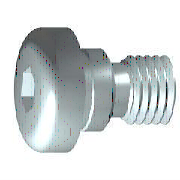
# Autodesk Inventor part: 100005
Saved by Autodesk Inventor 2020.1 (Build 241239000, 239)
## iProperties
Created: 2006-01-26
Part Number: 100005
Material: Steel, Mild
Description: Hexagon socket head shoulder screws
Document SubType Name: Modeling
Standard: ISO  7379
Designer: Kevin
Standard Revision: First edition 1983-10-01
Standards Organization: ISO
Language: en-US
Size Designation: 8  x 30
Categories: <MemberInstance><Categories><Category DisplayName="Fasteners" InternalName="e4da775c-781d-43d5-af7c-5136215cf5a6" Mnemonic="FSTN"><Category DisplayName="Bolts" InternalName="536e6df0-f778-49ac-b2f2-25c71d2aa0b2" Mnemonic="SCRW"><CategoryParameter DisplayName="Nominal Diameter" InternalName="8bbe3f8e-44cf-40a9-a251-3a6edc8168d6" Mnemonic="nomdia"/><CategoryParameter DisplayName="Nominal Length" InternalName="238ecbaf-3e6c-45dd-aa95-4068c8e0fd02" Mnemonic="nomlen"/><CategoryParameter DisplayName="Thread Series Designation" InternalName="87c5849c-b3a5-4c3e-9c9b-2feecef9be86" Mnemonic="thrserdsgn"/><CategoryParameter DisplayName="Thread Class" InternalName="ebc0d23b-2cc6-4d2a-b376-d52aae53bab6" Mnemonic="thrclss"/><CategoryParameter DisplayName="Thread Designation" InternalName="586d5e89-370a-4089-914f-0110033585c7" Mnemonic="thrdesign"/><CategoryParameter DisplayName="Thread Type" InternalName="b4bbb7bc-d6aa-4c9f-a9a9-4152b9f6fe49" Mnemonic="thrtype"/><CategoryParameter DisplayName="Threads per Unit" InternalName="bdc6e7d2-ffd0-4d9c-a173-16b95ebb912d" Mnemonic="thrperunit1"/><CategoryParameter DisplayName="Thread Pitch" InternalName="bb82302e-82d8-4176-8fc1-c5d7bb17d5ad" Mnemonic="pitch1"/><CategoryParameter DisplayName="Nominal Diameter Designation" InternalName="03caf894-eafd-4c09-a035-916ac084b87b" Mnemonic="nomdiadesig"/><Category DisplayName="Socket Head" InternalName="55e06bf3-7e58-486c-bbdc-745fcc60664d" Mnemonic="CLSCRW"><CategoryParameter DisplayName="Shank Diameter" InternalName="179dbae3-102f-48bb-85fe-1e3ecd34f7cc" Mnemonic="grpdia"/><CategoryParameter DisplayName="Grip Length" InternalName="52eab69f-422f-4795-9995-175a1b827e67" Mnemonic="grplen"/><CategoryParameter DisplayName="Thread Length" InternalName="3268731d-5f9a-4750-8b01-4a959c46fbf2" Mnemonic="thrlen"/><CategoryParameter DisplayName="Head Diameter" InternalName="46177176-dbdd-4a1b-aefd-4c60c45016af" Mnemonic="headdia"/><CategoryParameter DisplayName="Head Height" InternalName="99c92c4c-4a02-4ebe-9e64-948fb169e19e" Mnemonic="headh"/><CategoryParameter DisplayName="Type" InternalName="59a7e495-7a0c-4a5c-bdfd-c090c5f6e2db" Mnemonic="type"/><Category DisplayName="Shoulder" InternalName="90bdf7a4-4d26-46b5-8948-baa3e50baddb" Mnemonic="FTCLSCREW"><CategoryParameter DisplayName="Shank Length" InternalName="fd35b191-8e29-43b8-8902-775fde943ca0" Mnemonic="shnklen"/><CategoryParameter DisplayName="Shank Diameter" InternalName="3f11206c-57b2-4a53-88eb-c02e573d836e" Mnemonic="grpdia"/></Category></Category></Category></Category></Categories><FamilyTemplate Id="nf0093"><FamilyTemplateParameters><FamilyTemplateParameter ObjectType="kUserParameterObject" ValueType="xs:double" Id="1" ObjectReferenceKey="KOD"/><FamilyTemplateParameter ObjectType="kUserParameterObject" ValueType="xs:double" Id="2" ObjectReferenceKey="BDMM"/><FamilyTemplateParameter ObjectType="kUserParameterObject" ValueType="xs:double" Id="3" ObjectReferenceKey="FAWI3"/><FamilyTemplateParameter ObjectType="kUserParameterObject" ValueType="xs:double" Id="4" ObjectReferenceKey="FAWI2"/><FamilyTemplateParameter ObjectType="kUserParameterObject" ValueType="xs:double" Id="5" ObjectReferenceKey="BDM"/><FamilyTemplateParameter ObjectType="kUserParameterObject" ValueType="xs:double" Id="6" ObjectReferenceKey="SW"/><FamilyTemplateParameter ObjectType="kUserParameterObject" ValueType="xs:double" Id="7" ObjectReferenceKey="FAWI4"/><FamilyTemplateParameter ObjectType="kUserParameterObject" ValueType="xs:double" Id="8" ObjectReferenceKey="PTC"/><FamilyTemplateParameter ObjectType="kUserParameterObject" ValueType="xs:double" Id="9" ObjectReferenceKey="NLG"/><FamilyTemplateParameter ObjectType="kUserParameterObject" ValueType="xs:double" Id="10" ObjectReferenceKey="LOTI"/><FamilyTemplateParameter ObjectType="kUserParameterObject" ValueType="xs:double" Id="11" ObjectReferenceKey="BOR"/><FamilyTemplateParameter ObjectType="kUserParameterObject" ValueType="xs:double" Id="12" ObjectReferenceKey="GUL"/><FamilyTemplateParameter ObjectType="kUserParameterObject" ValueType="xs:double" Id="13" ObjectReferenceKey="SLG"/><FamilyTemplateParameter ObjectType="kUserParameterObject" ValueType="xs:double" Id="14" ObjectReferenceKey="THREADDIA"/><FamilyTemplateParameter ObjectType="kUserParameterObject" ValueType="xs:double" Id="15" ObjectReferenceKey="E0"/><FamilyTemplateParameter ObjectType="kUserParameterObject" ValueType="xs:double" Id="16" ObjectReferenceKey="TPU"/><FamilyTemplateParameter ObjectType="kUserParameterObject" ValueType="xs:double" Id="17" ObjectReferenceKey="TOA"/><FamilyTemplateParameter ObjectType="kUserParameterObject" ValueType="xs:double" Id="18" ObjectReferenceKey="SPD"/><FamilyTemplateParameter ObjectType="kUserParameterObject" ValueType="xs:double" Id="19" ObjectReferenceKey="PHH"/><FamilyTemplateParameter ObjectType="kUserParameterObject" ValueType="xs:double" Id="20" ObjectReferenceKey="ANG"/><FamilyTemplateParameter ObjectType="kUserParameterObject" ValueType="xs:double" Id="21" ObjectReferenceKey="NND"/><FamilyTemplateParameter ObjectType="kUserParameterObject" ValueType="xs:double" Id="22" ObjectReferenceKey="GD1"/><FamilyTemplateParameter ObjectType="kUserParameterObject" ValueType="xs:double" Id="23" ObjectReferenceKey="GEL"/><FamilyTemplateParameter ObjectType="kUserParameterObject" ValueType="xs:double" Id="24" ObjectReferenceKey="INTI"/><FamilyTemplateParameter ObjectType="kUserParameterObject" ValueType="xs:double" Id="25" ObjectReferenceKey="GAL2"/><FamilyTemplateParameter ObjectType="kUserParameterObject" ValueType="xs:double" Id="26" ObjectReferenceKey="GAL"/><FamilyTemplateParameter ObjectType="kUserParameterObject" ValueType="xs:double" Id="27" ObjectReferenceKey="KOH"/><FamilyTemplateParameter ObjectType="kPropertyObject" ValueType="xs:string" Id="100" ObjectReferenceKey="{32853F0F-3444-11D1-9E93-0060B03C1CA6}" SubObjectId="52"/><FamilyTemplateParameter ObjectType="kPropertyObject" ValueType="xs:string" Id="101" ObjectReferenceKey="{32853F0F-3444-11D1-9E93-0060B03C1CA6}" SubObjectId="49"/><FamilyTemplateParameter ObjectType="kPropertyObject" ValueType="xs:string" Id="102" ObjectReferenceKey="{32853F0F-3444-11D1-9E93-0060B03C1CA6}" SubObjectId="37"/><FamilyTemplateParameter ObjectType="kPropertyObject" ValueType="xs:string" Id="103" ObjectReferenceKey="{32853F0F-3444-11D1-9E93-0060B03C1CA6}" SubObjectId="47"/><FamilyTemplateParameter ObjectType="kPropertyObject" ValueType="xs:string" Id="104" ObjectReferenceKey="{32853F0F-3444-11D1-9E93-0060B03C1CA6}" SubObjectId="48"/><FamilyTemplateParameter ObjectType="kPropertyObject" ValueType="xs:string" Id="105" ObjectReferenceKey="{32853F0F-3444-11D1-9E93-0060B03C1CA6}" SubObjectId="5"/><FamilyTemplateParameter ObjectType="kPropertyObject" ValueType="xs:string" Id="106" ObjectReferenceKey="{32853F0F-3444-11D1-9E93-0060B03C1CA6}" SubObjectId="29"/><FamilyTemplateParameter ObjectType="kPropertyObject" ValueType="xs:string" Id="107" ObjectReferenceKey="{32853F0F-3444-11D1-9E93-0060B03C1CA6}" SubObjectId="20"/><FamilyTemplateParameter ObjectType="kPropertyObject" ValueType="xs:string" Id="108" ObjectReferenceKey="{B9600981-DEE8-4547-8D7C-E525B3A1727A}" SubObjectId="17"/><FamilyTemplateParameter ObjectType="kPropertyObject" ValueType="xs:string" Id="109" ObjectReferenceKey="{B9600981-DEE8-4547-8D7C-E525B3A1727A}" SubObjectId="19"/><FamilyTemplateParameter ObjectType="kPropertyObject" ValueType="xs:string" Id="110" ObjectReferenceKey="{B9600981-DEE8-4547-8D7C-E525B3A1727A}" SubObjectId="21"/><FamilyTemplateParameter ObjectType="kPropertyObject" ValueType="xs:string" Id="111" ObjectReferenceKey="{B9600981-DEE8-4547-8D7C-E525B3A1727A}" SubObjectId="9"/><FamilyTemplateParameter ObjectType="kPartDocumentObject" ValueType="xs:string" Id="112" ObjectReferenceKey="" SubObjectId="DisplayName"/><FamilyTemplateParameter ObjectType="kThreadFeatureObject" ValueType="xs:structure" Id="300" ObjectReferenceKey="1002000010000000e30a0000000000008000000000000000" SubObjectId="ThreadInfo"><FamilyTemplateParameter ValueType="xs:string" Id="301" SubObjectId="ThreadClass"/><FamilyTemplateParameter ValueType="xs:string" Id="302" SubObjectId="ThreadDesignation"/><FamilyTemplateParameter ValueType="xs:string" Id="303" SubObjectId="ThreadType"/></FamilyTemplateParameter><FamilyTemplateParameter ObjectType="kPartFeatureObject" ValueType="xs:string" Id="400" ObjectReferenceKey="10020000100000009f070000000000008000000000000000" SubObjectId="Name"/><FamilyTemplateParameter ObjectType="kPartFeatureObject" ValueType="xs:string" Id="401" ObjectReferenceKey="10020000100000004e080000000000008000000000000000" SubObjectId="Name"/><FamilyTemplateParameter ObjectType="kPartFeatureObject" ValueType="xs:string" Id="402" ObjectReferenceKey="10020000100000009d080000000000008000000000000000" SubObjectId="Name"/><FamilyTemplateParameter ObjectType="kPartFeatureObject" ValueType="xs:string" Id="403" ObjectReferenceKey="1002000010000000e30a0000000000008000000000000000" SubObjectId="Name"/><FamilyTemplateParameter ObjectType="kPartFeatureObject" ValueType="xs:string" Id="404" ObjectReferenceKey="1002000010000000ed080000000000008000000000000000" SubObjectId="Name"/><FamilyTemplateParameter ObjectType="kPartFeatureObject" ValueType="xs:string" Id="405" ObjectReferenceKey="100200001000000043090000000000008000000000000000" SubObjectId="Name"/><FamilyTemplateParameter ObjectType="kPartFeatureObject" ValueType="xs:string" Id="406" ObjectReferenceKey="10020000100000007b0b0000000000008000000000000000" SubObjectId="Name"/><FamilyTemplateParameter ObjectType="kPartFeatureObject" ValueType="xs:string" Id="407" ObjectReferenceKey="1002000010000000310c0000000000008000000000000000" SubObjectId="Name"/><FamilyTemplateParameter ObjectType="kPartFeatureObject" ValueType="xs:string" Id="408" ObjectReferenceKey="10020000100000001b000000000000008000000000000000" SubObjectId="Name"/><FamilyTemplateParameter ObjectType="kPartFeatureObject" ValueType="xs:string" Id="409" ObjectReferenceKey="1002000010000000c1070000000000008000000000000000" SubObjectId="Name"/><FamilyTemplateParameter ObjectType="kiMateDefinitionObject" ValueType="xs:string" Id="500" ObjectReferenceKey="040101001000000029cc8d7a704c7672ba90e38dc12e535a" SubObjectId="Name"/><FamilyTemplateParameter ObjectType="kiMateDefinitionObject" ValueType="xs:string" Id="501" ObjectReferenceKey="040101001000000013550299b947795b2766c691a833c807" SubObjectId="Name"/><FamilyTemplateParameter ObjectType="kiMateDefinitionObject" ValueType="xs:string" Id="502" ObjectReferenceKey="0401010010000000eced873f35484acdbce674909201d06c" SubObjectId="Name"/><FamilyTemplateParameter ObjectType="kiPartTableColumnObject" ValueType="xs:string" Id="503" ObjectReferenceKey="RID"/><FamilyTemplateParameter ObjectType="kiPartTableColumnObject" ValueType="xs:string" Id="504" ObjectReferenceKey="KLG"/><FamilyTemplateParameter ObjectType="kiPartTableColumnObject" ValueType="xs:string" Id="505" ObjectReferenceKey="THREADCLASSEXT"/><FamilyTemplateParameter ObjectType="kiPartTableColumnObject" ValueType="xs:string" Id="506" ObjectReferenceKey="SIZE_SEL"/><FamilyTemplateParameter ObjectType="kiPartTableColumnObject" ValueType="xs:string" Id="507" ObjectReferenceKey="THREADTYPE"/></FamilyTemplateParameters></FamilyTemplate><CategoryParameterMap><ParamToTemplateMap><ParamToTemplate CategoryParameter="//CategoryParameter[@InternalName='3f11206c-57b2-4a53-88eb-c02e573d836e']" TemplateParameter="5"/><ParamToTemplate CategoryParameter="//CategoryParameter[@InternalName='2675968c-4ce5-49e0-a4f5-552d29089031']" TemplateParameter="100"/><ParamToTemplate CategoryParameter="//CategoryParameter[@InternalName='8b46a4cc-9585-4fed-90c3-899f57e09a73']" TemplateParameter="110"/><ParamToTemplate CategoryParameter="//CategoryParameter[@InternalName='3268731d-5f9a-4750-8b01-4a959c46fbf2']" TemplateParameter="23"/><ParamToTemplate CategoryParameter="//CategoryParameter[@InternalName='52eab69f-422f-4795-9995-175a1b827e67']" TemplateParameter="504"/><ParamToTemplate CategoryParameter="//CategoryParameter[@InternalName='46177176-dbdd-4a1b-aefd-4c60c45016af']" TemplateParameter="1"/><ParamToTemplate CategoryParameter="//CategoryParameter[@InternalName='99c92c4c-4a02-4ebe-9e64-948fb169e19e']" TemplateParameter="27"/><ParamToTemplate CategoryParameter="//CategoryParameter[@InternalName='818a152a-d3c3-49ca-80ee-df7d91421b8e']" TemplateParameter="107"/><ParamToTemplate CategoryParameter="//CategoryParameter[@InternalName='238ecbaf-3e6c-45dd-aa95-4068c8e0fd02']" TemplateParameter="9"/><ParamToTemplate CategoryParameter="//CategoryParameter[@InternalName='8bbe3f8e-44cf-40a9-a251-3a6edc8168d6']" TemplateParameter="21"/><ParamToTemplate CategoryParameter="//CategoryParameter[@InternalName='016b6077-bfbe-49bd-92c9-d8d59c39c941']" TemplateParameter="105"/><ParamToTemplate CategoryParameter="//CategoryParameter[@InternalName='bb82302e-82d8-4176-8fc1-c5d7bb17d5ad']" TemplateParameter="8"/><ParamToTemplate CategoryParameter="//CategoryParameter[@InternalName='8e5e0294-fc51-4c8f-b3d7-003dc5ed94f6']" TemplateParameter="503"/><ParamToTemplate CategoryParameter="//CategoryParameter[@InternalName='03caf894-eafd-4c09-a035-916ac084b87b']" TemplateParameter="506"/><ParamToTemplate CategoryParameter="//CategoryParameter[@InternalName='fd35b191-8e29-43b8-8902-775fde943ca0']" TemplateParameter="13"/><ParamToTemplate CategoryParameter="//CategoryParameter[@InternalName='ebc0d23b-2cc6-4d2a-b376-d52aae53bab6']" TemplateParameter="505"/><ParamToTemplate CategoryParameter="//CategoryParameter[@InternalName='586d5e89-370a-4089-914f-0110033585c7']" TemplateParameter="302"/><ParamToTemplate CategoryParameter="//CategoryParameter[@InternalName='b4bbb7bc-d6aa-4c9f-a9a9-4152b9f6fe49']" TemplateParameter="507"/><ParamToTemplate CategoryParameter="//CategoryParameter[@InternalName='bdc6e7d2-ffd0-4d9c-a173-16b95ebb912d']" TemplateParameter="16"/></ParamToTemplateMap></CategoryParameterMap></MemberInstance>
Density: 7.85 g/cm^3
Appearance: Steel
Mass: 19.0283 g
Volume: 2.42398 cm^3
Author: Kevin
Autodesk Inventor part; units mm, degrees
ref_plane "YZ Plane" through (0, 0, 0) normal (1, 0, 0) x (0, 1, 0)
ref_plane "XZ Plane" through (0, 0, 0) normal (0, 1, 0) x (-1, 0, 0)
sketch "Sketch1" plane through (0, 0, 0) normal (0, 0, 1) x (1, 0, 0)
  line L0 (-0.8667, 0) -> (41.25, 0)
  line L1 (41.25, 0) -> (41.25, 3)
  line L2 (41.25, 3) -> (30, 3)
  line L3 (30, 3) -> (30, 4)
  line L4 (30, 4) -> (0, 4)
  line L5 (0, 4) -> (0, 6.5)
  line L6 (0, 6.5) -> (-5.5, 6.5)
  line L7 (-5.5, 6.5) -> (-5.5, 2.3094)
  line L8 (-5.5, 2.3094) -> (-2.2, 2.3094)
  line L9 (-2.2, 2.3094) -> (-0.8667, 0)
  line L10 (-10.175, 0) -> (55.275, 0) projected
  line L11 (0, -0.65) -> (0, 8.45) projected
  line L12 (0, 3.71) -> (2.5, 3.71)
  line L13 (2.5, 3.71) -> (2.79, 4)
  line L14 (30, 3) -> (30, 2.3865)
  line L15 (30, 2.3865) -> (30.6134, 2.3865)
  line L16 (30.6134, 2.3865) -> (31.676, 3)
  line L17 (0, 3.71) -> (0, 4)
  dimension "d0" = 6
  dimension "d1" = 8
  dimension "d2" = 13
  dimension "d3" = 4.6188
  dimension "d5" = 11.25
  dimension "d6" = 5.5
  dimension "d7" = 3.3
  dimension "d8" = 60
  dimension "d9" = 41.25
  dimension "d18" = 2.5
  dimension "d19" = 45
  dimension "d20" = 7.42
  dimension "d21" = 4.7731
  dimension "d22" = 30
  dimension "d23" = 0.6135
  constraints: 32 end point, 7 parallel, 5 perpendicular, 3 point on line, 2 collinear, 1 horizontal
  measures "d0" diameter of L2 L0
  measures "d1" diameter of L4 L0
  measures "d2" diameter of L6 L0
  measures "d3" diameter of L8 L0
  measures "d5" distance between parallel lines of L3 L1
  measures "d6" distance between parallel lines of L5 L7
  measures "d7" distance from line of L8.end L7
  measures "d8" angle of L9 L0
  measures "d9" distance between parallel lines of L1 L5
  measures "d18" distance from line of L12.end L11
  measures "d19" angle of L13 L4
  measures "d20" diameter of L12 L0
  measures "d21" diameter of L15 L0
  measures "d22" angle of L16 L15
  measures "d23" distance of L14.end L15.end
revolve "Body" add sketch "Sketch1" angle 360 about axis through (-0.8667, 0, 0) along (1, 0, 0)
sketch "Sketch2" plane through (-5.5, 0, 0) normal (-1, 0, 0) x (0, 0, 1)
  circle A0 centre (0, 0) radius 2.3094 projected
  line L0 (0, 2.3094) -> (2, 1.1547)
  line L1 (2, 1.1547) -> (2, -1.1547)
  line L2 (2, -1.1547) -> (0, -2.3094)
  line L3 (0, -2.3094) -> (-2, -1.1547)
  line L4 (-2, -1.1547) -> (-2, 1.1547)
  line L5 (-2, 1.1547) -> (0, 2.3094)
  point P0 (0, 0)
  constraints: 12 end point, 1 coincident, 1 vertical, 1 vertical alignment, 12 other
extrude "Slot" add sketch "Sketch2" against normal up to next contours A0 L1 | L0 A0 | A0 L2 | L5 A0 | A0 L3 | L4 A0
fillet "Fillet1" radius 2.3622 1 edges at (-5.5, -6.5, 0)
thread "Thread" size "M6x1" class "6g" standard "ISO Metric profile" length 11.25
chamfer "Chamfer1" distance 0.6135 distance2 0.6135 1 edges at (41.25, -3, 0) measured on face at (41.25, 1, 0)
chamfer "Chamfer2" distance 1 angle 1 1 edges at (30, -4, 0) measured on face at (30, 3.5989, -0.5584)
revolve "Groove1" cut sketch "Sketch1" angle 360 about axis through (-0.8667, 0, 0) along (1, 0, 0) contours L11 L4 L13 L12
revolve "Groove2" cut sketch "Sketch1" angle 360 about axis through (-0.8667, 0, 0) along (1, 0, 0) contours L16 L15 L14 L2
ref_plane "Work Plane1" through (15, 0, 0) normal (0, 0, 1) x (1, 0, 0)
equation "\"d0\" = NND"
equation "\"d1\" = BDM"
equation "\"d2\" = KOD"
equation "\"d3\" = 1.1547 * SW"
equation "\"d5\" = GEL"
equation "\"d6\" = KOH"
equation "\"d7\" = INTI + LOTI"
equation "\"d8\" = 0.5 * ANG"
equation "\"d9\" = NLG"
equation "\"d18\" = GAL2"
equation "\"d19\" = FAWI4"
equation "\"d20\" = BDMM"
equation "\"d21\" = GD1"
equation "\"d22\" = FAWI2"
equation "\"d23\" = GAL"
equation "\"d13\" = RR"
equation "\"d25\" = GEL"
equation "\"d14\" = -0.5 * SPD + 0.5 * NND"
equation "\"d15\" = GUL"
equation "\"d16\" = -0.5 * NND + 0.5 * BDM"
equation "\"d32\" = -0.5 * NND + 0.5 * BDM"
equation "\"NND\" = 6"
equation "\"NLG\" = 41.25"
equation "\"GEL\" = 11.25"
equation "\"KOD\" = 13"
equation "\"KOH\" = 5.5"
equation "\"INTI\" = 3.3"
equation "\"GAL\" = 0.61345 * PTC"
equation "\"GUL\" = 0.61345 * PTC"
equation "\"SPD\" = NND - 1.2269 * PTC"
equation "\"BDM\" = 8"
equation "\"ANG\" = 120deg"
equation "\"FAWI2\" = 30deg"
equation "\"FAWI3\" = 89deg"
equation "\"FAWI4\" = 45deg"
equation "\"RR\" = 2.3622"
equation "\"SW\" = 4"
equation "\"BDMM\" = 7.42"
equation "\"GAL2\" = 2.5"
equation "\"LOTI\" = 0"
equation "\"GD1\" = THREADDIA - 1.2269 * PTC"
equation "\"PTC\" = 1"
equation "\"BOR\" = 4"
equation "\"THREADDIA\" = 6"
equation "\"E0\" = 1.155 * SW"
equation "\"TOA\" = 30deg"
equation "\"PHH\" = 0.55"
body "Solid1"
